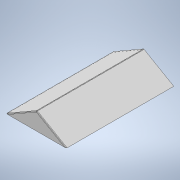
# Autodesk Inventor part: tapa_marco
Saved by Autodesk Inventor 2021 (Build 250183000, 183)
## iProperties
Created: 2021-11-09
Part Number: tapa_marco
Material: Genérico
Document SubType Name: Modeling
Designer: arthu
Density: 1 g/cm^3
Appearance: Valor por defecto
Author: arthu
Autodesk Inventor part; units mm, degrees
ref_plane "YZ Plane" through (0, 0, 0) normal (1, 0, 0) x (0, 1, 0)
ref_plane "XZ Plane" through (0, 0, 0) normal (0, 1, 0) x (-1, 0, 0)
ref_plane "XY Plane" through (0, 0, 0) normal (0, 0, 1) x (1, 0, 0)
sketch "Boceto1" plane through (0, 0, 0) normal (0, 0, 1) x (1, 0, 0)
  line L0 (-146.2, 146.2) -> (146.2, 146.2)
  line L1 (-146.2, 146.2) -> (0, 230.6086)
  line L2 (-146.2, 146.2) -> (32.5033, 146.2) construction
  line L3 (0, 230.6086) -> (146.2, 146.2)
  point P0 (0, 0)
  dimension "d2" = 30
  constraints: 8 end point, 1 horizontal
  measures "d2" angle of L2 L1
extrude "Extrusión1" add sketch "Boceto1" along normal blind 522.4
shell "Vaciado1" thickness 1.2 removed faces 1 at (-48.7333, 146.2, 174.1333)
fillet "Empalme1" radius 4 5 edges at (0, 230.6086, 261.2) (-73.1, 188.4043, 522.4) (73.1, 188.4043, 522.4) (71.9, 187.7115, 1.2) (-71.9, 187.7115, 1.2)
